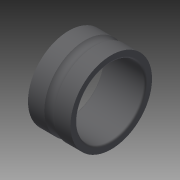
# Autodesk Inventor part: MF74ZZ Inner Ring
Saved by Autodesk Inventor 2014 SP2 (Build 180246200, 246)
## iProperties
Created: 2019-11-12
Part Number: MF74ZZ Inner Ring
Material: Generic
Catalog Web Link: www.cadenas.de
Description: shielded_type_zz_zzs_IR-
Vendor: NSK_RB
Document SubType Name: Modeling
Designer: psadmin
Manufacturer: NSK_RB
Mass: 0.0131956 g
Surface Area: 0.795434 cm^2
Volume: 0.0131956 cm^3
Density: 1 g/cm^3
Appearance: PSOLRGB-128-128-128
Category: PARTsolutions
Company: NSK_RB
Title: MF74ZZ Inner Ring
Author: Cadenas PARTsolutions
PSOL_IDENT_0: {$CADENAS_DATA\23d-libs\nsk_rb\roller_bearings\deep_groove_bb\exstra_small_miniatur_bb\metric_design
PSOL_IDENT_1: _with_flange\shielded_type_zz_zzs_ir_1.prj},192 {VTYP=3D},{NB=MF74ZZ Inner Ring},{LINA=MF74ZZ Inner
PSOL_IDENT_2: Ring},{NN=shielded_type_zz_zzs_IR},{DATE=16.01.2019 01:41:16},{GEOMDATE=04.01.2008 00:00:00},{VERSIO
PSOL_IDENT_3: N=},{LINEID=290},{WBVAR=},{WBNUMERIC=}  {NB=MF74ZZ Inner Ring},{LINA=MF74ZZ Inner Ring},{KT=DUMMY},{
PSOL_IDENT_4: IDNR=},{STAN=},{ORDER=MF74ZZ},{SD=4.0},{X=4.0},{D=7},{DD=7},{DD1=0.0},{D2=8.2},{DD2=8.2},{B=0.0},{B1=
PSOL_IDENT_5: 2.5},{CC1=0.0},{C2=0.6},{CC2=0.6},{R=0.00},{R1=0.10},{DI1=4.80},{DI2=4.80},{SDE1=6.00},{SDE2=6.30},{
PSOL_IDENT_6: CR1=255},{COR1=107},{CR2=26},{COR2=11.0},{LG=60000},{LO=67000},{DA=0.0},{DB=4.8},{RA=0.00},{RB=0.10}
PSOL_IDENT_7: ,{MASS=0.35},{SC=1},{N=14}
NN: shielded_type_zz_zzs_IR
NB: MF74ZZ Inner Ring
NBSYN: $ORDER. Inner Ring
LINA: MF74ZZ Inner Ring
ORDER: MF74ZZ
SD: 4
X: 4
D: 7
DD: 7
DD1: 0
D2: 8.2
DD2: 8.2
B: 0
B1: 2.5
CC1: 0
C2: 0.6
CC2: 0.6
R: 0
R1: 0.1
DI1: 4.8
DI2: 4.8
SDE1: 6
SDE2: 6.3
CR1: 255
COR1: 107
CR2: 26
COR2: 11
LG: 60000
LO: 67000
DA: 0
DB: 4.8
RA: 0
RB: 0.1
MASS: 0.35
SC: 1
SUPPLIER: NSK_RB
ARTICLENO: MF74ZZ Inner Ring
BOMINFO: MF74ZZ Inner Ring
CREATOR: CADENAS GmbH
Autodesk Inventor part; units mm, degrees
sketch "Sketch_1" plane through (0, 0, 0) normal (0, 0, 1) x (1, 0, 0)
  line L0 (2.5, 0) -> (0, 0)
  arc A0 (0, 2.1) -> (0.1, 2) centre (0.1, 2.1) ccw
  line L1 (0.1, 2) -> (2.4, 2)
  arc A1 (2.4, 2) -> (2.5, 2.1) centre (2.4, 2.1) ccw
  line L2 (2.5, 2.1) -> (2.5, 2.4)
  line L3 (2.5, 2.4) -> (1.5328, 2.4)
  arc A2 (0.9672, 2.4) -> (1.5328, 2.4) centre (1.25, 2.75) ccw
  line L4 (0.9672, 2.4) -> (0, 2.4)
  line L5 (0, 2.4) -> (0, 2.1)
  constraints: 12 end point, 6 point on circle, 3 centre point
revolve "Revolution1" add sketch "Sketch_1" angle 360 about axis through (2.5, 0, 0) along (1, 0, 0)
ref_plane "ip_st_1_1_XY" through (1.25, 2.75, 0) normal (1, 0, 0) x (0, 0, -1)
ref_plane "ip_st_1_1_YZ" through (1.25, 2.75, 0) normal (0, 0, -1) x (0, 1, 0)
ref_plane "ip_st_1_1_ZX" through (1.25, 2.75, 0) normal (0, 1, 0) x (1, 0, 0)
ref_plane "ip_st_1_10_XY" through (1.25, -1.7146, -2.15) normal (1, 0, 0) x (0, 0, -1)
ref_plane "ip_st_1_10_YZ" through (1.25, -1.7146, -2.15) normal (0, 0, -1) x (0, 1, 0)
ref_plane "ip_st_1_10_ZX" through (1.25, -1.7146, -2.15) normal (0, 1, 0) x (1, 0, 0)
ref_plane "ip_st_1_11_XY" through (1.25, -0.6119, -2.6811) normal (1, 0, 0) x (0, 0, -1)
ref_plane "ip_st_1_11_YZ" through (1.25, -0.6119, -2.6811) normal (0, 0, -1) x (0, 1, 0)
ref_plane "ip_st_1_11_ZX" through (1.25, -0.6119, -2.6811) normal (0, 1, 0) x (1, 0, 0)
ref_plane "ip_st_1_12_XY" through (1.25, 0.6119, -2.6811) normal (1, 0, 0) x (0, 0, -1)
ref_plane "ip_st_1_12_YZ" through (1.25, 0.6119, -2.6811) normal (0, 0, -1) x (0, 1, 0)
ref_plane "ip_st_1_12_ZX" through (1.25, 0.6119, -2.6811) normal (0, 1, 0) x (1, 0, 0)
ref_plane "ip_st_1_13_XY" through (1.25, 1.7146, -2.15) normal (1, 0, 0) x (0, 0, -1)
ref_plane "ip_st_1_13_YZ" through (1.25, 1.7146, -2.15) normal (0, 0, -1) x (0, 1, 0)
ref_plane "ip_st_1_13_ZX" through (1.25, 1.7146, -2.15) normal (0, 1, 0) x (1, 0, 0)
ref_plane "ip_st_1_14_XY" through (1.25, 2.4777, -1.1932) normal (1, 0, 0) x (0, 0, -1)
ref_plane "ip_st_1_14_YZ" through (1.25, 2.4777, -1.1932) normal (0, 0, -1) x (0, 1, 0)
ref_plane "ip_st_1_14_ZX" through (1.25, 2.4777, -1.1932) normal (0, 1, 0) x (1, 0, 0)
ref_plane "ip_st_1_2_XY" through (1.25, 2.4777, 1.1932) normal (1, 0, 0) x (0, 0, -1)
ref_plane "ip_st_1_2_YZ" through (1.25, 2.4777, 1.1932) normal (0, 0, -1) x (0, 1, 0)
ref_plane "ip_st_1_2_ZX" through (1.25, 2.4777, 1.1932) normal (0, 1, 0) x (1, 0, 0)
ref_plane "ip_st_1_3_XY" through (1.25, 1.7146, 2.15) normal (1, 0, 0) x (0, 0, -1)
ref_plane "ip_st_1_3_YZ" through (1.25, 1.7146, 2.15) normal (0, 0, -1) x (0, 1, 0)
ref_plane "ip_st_1_3_ZX" through (1.25, 1.7146, 2.15) normal (0, 1, 0) x (1, 0, 0)
ref_plane "ip_st_1_4_XY" through (1.25, 0.6119, 2.6811) normal (1, 0, 0) x (0, 0, -1)
ref_plane "ip_st_1_4_YZ" through (1.25, 0.6119, 2.6811) normal (0, 0, -1) x (0, 1, 0)
ref_plane "ip_st_1_4_ZX" through (1.25, 0.6119, 2.6811) normal (0, 1, 0) x (1, 0, 0)
ref_plane "ip_st_1_5_XY" through (1.25, -0.6119, 2.6811) normal (1, 0, 0) x (0, 0, -1)
ref_plane "ip_st_1_5_YZ" through (1.25, -0.6119, 2.6811) normal (0, 0, -1) x (0, 1, 0)
ref_plane "ip_st_1_5_ZX" through (1.25, -0.6119, 2.6811) normal (0, 1, 0) x (1, 0, 0)
ref_plane "ip_st_1_6_XY" through (1.25, -1.7146, 2.15) normal (1, 0, 0) x (0, 0, -1)
ref_plane "ip_st_1_6_YZ" through (1.25, -1.7146, 2.15) normal (0, 0, -1) x (0, 1, 0)
ref_plane "ip_st_1_6_ZX" through (1.25, -1.7146, 2.15) normal (0, 1, 0) x (1, 0, 0)
ref_plane "ip_st_1_7_XY" through (1.25, -2.4777, 1.1932) normal (1, 0, 0) x (0, 0, -1)
ref_plane "ip_st_1_7_YZ" through (1.25, -2.4777, 1.1932) normal (0, 0, -1) x (0, 1, 0)
ref_plane "ip_st_1_7_ZX" through (1.25, -2.4777, 1.1932) normal (0, 1, 0) x (1, 0, 0)
ref_plane "ip_st_1_8_XY" through (1.25, -2.75, 0) normal (1, 0, 0) x (0, 0, -1)
ref_plane "ip_st_1_8_YZ" through (1.25, -2.75, 0) normal (0, 0, -1) x (0, 1, 0)
ref_plane "ip_st_1_8_ZX" through (1.25, -2.75, 0) normal (0, 1, 0) x (1, 0, 0)
ref_plane "ip_st_1_9_XY" through (1.25, -2.4777, -1.1932) normal (1, 0, 0) x (0, 0, -1)
ref_plane "ip_st_1_9_YZ" through (1.25, -2.4777, -1.1932) normal (0, 0, -1) x (0, 1, 0)
ref_plane "ip_st_1_9_ZX" through (1.25, -2.4777, -1.1932) normal (0, 1, 0) x (1, 0, 0)
ref_plane "ip_st_1a_XY" through (0, 0, 0) normal (1, 0, 0) x (0, 0, -1)
ref_plane "ip_st_1a_YZ" through (0, 0, 0) normal (0, 0, -1) x (0, 1, 0)
ref_plane "ip_st_1a_ZX" through (0, 0, 0) normal (0, 1, 0) x (1, 0, 0)
ref_plane "ip_st_2a_XY" through (0.1562, 0, 0) normal (1, 0, 0) x (0, 0, -1)
ref_plane "ip_st_2a_YZ" through (0.1562, 0, 0) normal (0, 0, -1) x (0, 1, 0)
ref_plane "ip_st_2a_ZX" through (0.1562, 0, 0) normal (0, 1, 0) x (1, 0, 0)
body "Solid1"
